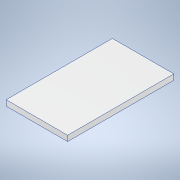
# Autodesk Inventor part: BELT WOOD SUPPORT
Saved by Autodesk Inventor 2021 (Build 250183000, 183)
## iProperties
Created: 2021-07-27
Part Number: BELT WOOD SUPPORT
Material: Aluminum 6061
Document SubType Name: Modeling
Designer: HP
Density: 2.7 g/cm^3
Appearance: Aluminum - Flat
Author: HP
Autodesk Inventor part; units mm, degrees
ref_plane "YZ Plane" through (0, 0, 0) normal (1, 0, 0) x (0, 1, 0)
ref_plane "XZ Plane" through (0, 0, 0) normal (0, 1, 0) x (-1, 0, 0)
ref_plane "XY Plane" through (0, 0, 0) normal (0, 0, 1) x (1, 0, 0)
sketch "Sketch1" plane through (0, 0, 0) normal (1, 0, 0) x (0, 1, 0)
  line L0 (0, 0) -> (-13.716, 0)
  line L1 (-13.716, 0) -> (-13.716, -263.1948)
  line L2 (-13.716, -263.1948) -> (0, -263.1948)
  line L3 (0, -263.1948) -> (0, 0)
  dimension "d0" = 13.716
  dimension "d1" = 263.1948
  constraints: 8 end point, 2 parallel, 1 horizontal, 1 perpendicular
  measures "d0" distance of L2.end L1.end
  measures "d1" distance of L1.end L0.end
extrude "Extrusion1" add sketch "Sketch1" along normal blind 152.4
body "Solid1"
